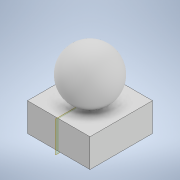
# Autodesk Inventor part: queen
Saved by Autodesk Inventor 2021 (Build 250183000, 183)
## iProperties
Created: 2021-01-12
Part Number: queen
Material: Generic
Document SubType Name: Modeling
Designer: Luke Kamols
Density: 1 g/cm^3
Appearance: Default
Author: Luke Kamols
Autodesk Inventor part; units mm, degrees
ref_plane "YZ Plane" through (0, 0, 0) normal (1, 0, 0) x (0, 1, 0)
ref_plane "XZ Plane" through (0, 0, 0) normal (0, 1, 0) x (-1, 0, 0)
ref_plane "XY Plane" through (0, 0, 0) normal (0, 0, 1) x (1, 0, 0)
sketch "Sketch6" plane through (0, 0, 0) normal (0, 1, 0) x (-1, 0, 0)
  line L0 (0, 0) -> (22, 0)
  line L1 (22, 0) -> (22, -22)
  line L2 (22, -22) -> (0, -22)
  line L3 (0, -22) -> (0, 0)
  dimension "d18" = 22
  dimension "d19" = 22
  constraints: 8 end point, 2 parallel, 1 horizontal, 1 perpendicular
  measures "d18" distance of L1.end L2.end
  measures "d19" distance of L0.end L1.end
extrude "Extrusion3" add sketch "Sketch6" along normal blind 10
ref_plane "Work Plane1" through (-11, 0, -22) normal (-1, 0, 0) x (0, 0, 1)
sketch "Sketch8" plane through (-11, 0, -22) normal (-1, 0, 0) x (0, 0, 1)
  line L0 (0, 10) -> (22, 10) projected
  line L1 (11, 10) -> (11, 18)
  circle A0 centre (11, 18) radius 9
  line L2 (11.0985, 9.0005) -> (10.9015, 26.9995)
  point P0 (22, 0)
  dimension "d30" = 8
  dimension "d31" = 18
  constraints: 4 end point, 2 midpoint, 2 point on circle, 1 centre point, 1 coincident, 1 vertical
  measures "d30" distance of L1.start L1.end
  measures "d31" diameter of A0
revolve "Revolution2" add sketch "Sketch8" angle 360 about axis through (-11, 9.0005, -10.9015) along (0, 0.9999401, -0.0109435) picked at (12.4036, 12.6667) picked at (13.3498, 9.8198) contours A0 L0 L2 | L2 L0 A0
body "Solid3"
